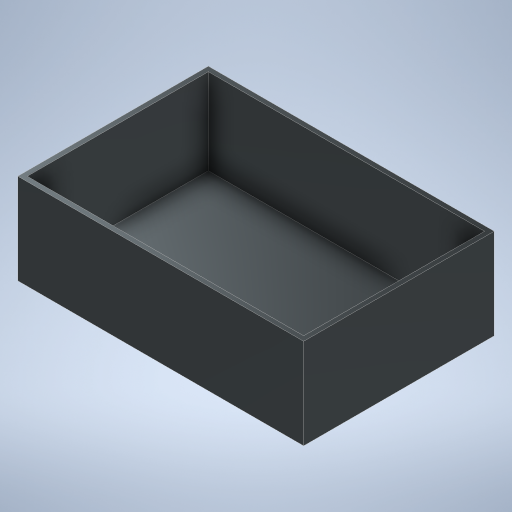
# Autodesk Inventor part: Box442
Saved by Autodesk Inventor 2024 (Build 280153000, 153)
## iProperties
Created: 2023-11-19
Part Number: Box442
Material: Generic
Document SubType Name: Modeling
Designer: nickiverson
Density: 1 g/cm^3
Appearance: Fine Textured - Black
Author: nickiverson
Autodesk Inventor part; units mm, degrees
ref_plane "YZ Plane" through (0, 0, 0) normal (1, 0, 0) x (0, 1, 0)
ref_plane "XZ Plane" through (0, 0, 0) normal (0, 1, 0) x (-1, 0, 0)
ref_plane "XY Plane" through (0, 0, 0) normal (0, 0, 1) x (1, 0, 0)
sketch "Sketch1" plane through (0, 0, 0) normal (0, 1, 0) x (-1, 0, 0)
  line L0 (0, 0) -> (-152.4, 0)
  line L1 (-152.4, 0) -> (-152.4, -101.6)
  line L2 (-152.4, -101.6) -> (0, -101.6)
  line L3 (0, -101.6) -> (0, 0)
  dimension "d0" = 152.4
  dimension "d1" = 101.6
  constraints: 8 end point, 2 parallel, 1 horizontal, 1 perpendicular
  measures "d0" distance of L2.end L1.end
  measures "d1" distance of L1.end L0.end
extrude "Extrusion1" add sketch "Sketch1" along normal blind 50.8
sketch "Sketch2" plane through (0, 50.8, 0) normal (0, 1, 0) x (1, 0, 0)
  line L0 (152.4, 101.6) -> (0, 101.6) projected
  line L1 (0, 0) -> (152.4, 0)
  line L2 (152.4, 0) -> (152.4, 101.6)
  line L3 (152.4, 101.6) -> (0, 101.6)
  line L4 (0, 101.6) -> (0, 0)
  line L5 (2.54, 2.54) -> (149.86, 2.54)
  line L6 (149.86, 2.54) -> (149.86, 99.06)
  line L7 (149.86, 99.06) -> (2.54, 99.06)
  line L8 (2.54, 99.06) -> (2.54, 2.54)
  dimension "d5" = 2.54
  constraints: 16 end point, 4 parallel, 2 perpendicular, 1 horizontal, 3 other
  measures "d5" distance between parallel lines of L4 L8
extrude "Extrusion2" cut sketch "Sketch2" against normal blind 48.26 contours L8 L7 L6 L5
sketch "Sketch4" plane through (152.4, 0, 0) normal (1, 0, 0) x (0, 0, -1)
  line L0 (101.6, 50.8) -> (0, 50.8) projected
  line L1 (0, 50.8) -> (101.6, 50.8)
  line L2 (101.6, 50.8) -> (101.6, 48.26)
  line L3 (101.6, 48.26) -> (0, 48.26)
  line L4 (0, 48.26) -> (0, 50.8)
  point P0 (0, 0)
  dimension "d8" = 101.6
  dimension "d9" = 2.54
  constraints: 8 end point, 2 parallel, 1 horizontal, 1 perpendicular
  measures "d8" distance of L2.end L3.end
  measures "d9" distance of L1.end L2.end
extrude "Extrusion3" cut sketch "Sketch4" against normal blind 156.5275
body "Solid1"
